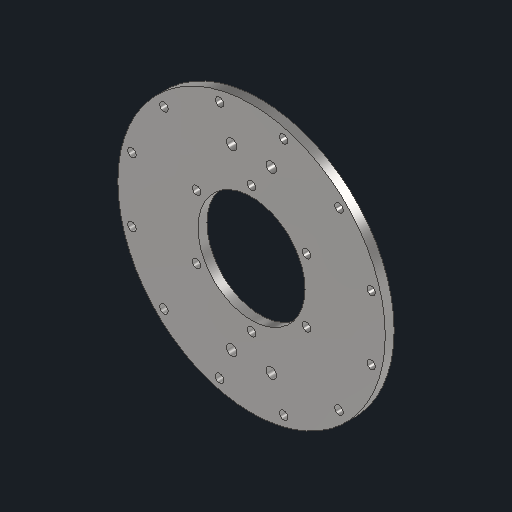
# Autodesk Inventor part: scara-plate1
Saved by Autodesk Inventor 2022 (Build 260153000, 153)
## iProperties
Created: 2021-10-10
Part Number: scara-plate1
Material: 鋼、炭素鋼
Document SubType Name: Sheet Metal
Designer: Yuta Kage
Density: 7.85 g/cm^3
Sheet Metal Rule: Default
Appearance: 半つや出し
Description: 在庫有
Author: Yuta Kage
Autodesk Inventor part; units mm, degrees
ref_plane "YZ Plane" through (0, 0, 0) normal (1, 0, 0) x (0, 1, 0)
ref_plane "XZ Plane" through (0, 0, 0) normal (0, 1, 0) x (-1, 0, 0)
ref_plane "XY Plane" through (0, 0, 0) normal (0, 0, 1) x (1, 0, 0)
sketch "スケッチ1" plane through (0, 0, 0) normal (0, 0, 1) x (1, 0, 0)
  line L0 (-20, -100) -> (20, -100)
  circle A0 centre (0, 0) radius 67.5
  dimension "d47" = 135
  constraints: 2 end point, 1 centre point, 1 coincident, 1 horizontal
  measures "d47" diameter of A0
extrude "プレート1" add sketch "スケッチ1" along normal blind 4.5
sketch "スケッチ2" plane through (0, 0, 4.5) normal (0, 0, 1) x (1, 0, 0)
  circle A0 centre (0, 0) radius 62.5
  point P0 (-44.1942, -44.1942)
  point P1 (-16.1762, -60.3704)
  point P2 (16.1762, -60.3704)
  point P3 (44.1942, -44.1942)
  point P4 (60.3704, -16.1762)
  point P5 (60.3704, 16.1762)
  point P6 (44.1942, 44.1942)
  point P7 (16.1762, 60.3704)
  point P8 (-16.1762, 60.3704)
  point P9 (-44.1942, 44.1942)
  point P10 (-60.3704, 16.1762)
  point P11 (-60.3704, -16.1762)
  dimension "d5" = 125
  dimension "d8" = 360
  dimension "d51" = 0
  constraints: 1 coincident, 16 other
  measures "d51" vertical distance of point (16.176, 60.37) point (-16.176, 60.37)
hole "穴1" at (-60.3704, -16.1762, 4.5) at (-60.3704, 16.1762, 4.5) at (-44.1942, 44.1942, 4.5) at (-16.1762, 60.3704, 4.5) at (16.1762, 60.3704, 4.5) at (44.1942, 44.1942, 4.5) at (60.3704, 16.1762, 4.5) at (60.3704, -16.1762, 4.5) at (44.1942, -44.1942, 4.5) at (16.1762, -60.3704, 4.5) at (-16.1762, -60.3704, 4.5) at (-44.1942, -44.1942, 4.5) direction (0, 0, -1) diameter 4.3 end through all clearance for "Socket Head Cap Screw" size "M4" standard "Ansi Metric M Profile"
sketch "スケッチ3" plane through (0, 0, 4.5) normal (0, 0, 1) x (1, 0, 0)
  circle A0 centre (0, 0) radius 27
  dimension "d18" = 54
  constraints: 1 centre point, 1 coincident
  measures "d18" diameter of A0
extrude "押し出し1" cut sketch "スケッチ3" against normal blind 10
sketch "スケッチ4" plane through (0, 0, 4.5) normal (0, 0, 1) x (1, 0, 0)
  line L0 (10, -45) -> (-10, -45)
  line L1 (-10, -45) -> (-10, 45)
  line L2 (-10, 45) -> (10, 45)
  line L3 (10, 45) -> (10, -45)
  line L4 (10, -45) -> (-10, 45) construction
  line L5 (-10, -45) -> (10, 45) construction
  circle A0 centre (0, 0) radius 45.5
  point P0 (0, 0)
  point P1 (0, 0)
  dimension "d21" = 20
  dimension "d46" = 91
  dimension "d48" = 90
  constraints: 12 end point, 4 midpoint, 3 coincident, 2 parallel, 1 centre point, 1 horizontal, 1 perpendicular
  measures "d21" distance of L1.end L2.end
  measures "d46" diameter of A0
  measures "d48" distance of L2.end L0.start
hole "穴2" at (-10, 45, 4.5) at (10, 45, 4.5) at (-10, -45, 4.5) at (10, -45, 4.5) direction (0, 0, -1) diameter 5.3 end through all clearance for "Socket Head Cap Screw" size "M5" standard "Ansi Metric M Profile"
sketch "スケッチ5" plane through (0, 0, 4.5) normal (0, 0, 1) x (1, 0, 0)
  circle A0 centre (0, 0) radius 32
  point P0 (0, 32)
  point P1 (-27.7128, 16)
  point P2 (-27.7128, -16)
  point P3 (0, -32)
  point P4 (27.7128, -16)
  point P5 (27.7128, 16)
  dimension "d33" = 64
  dimension "d36" = 360
  dimension "d49" = 0
  constraints: 1 coincident, 1 vertical alignment, 9 other
  measures "d49" horizontal distance of point (0, -32) point (0, 32)
hole "穴3" at (0, 32, 4.5) at (-27.7128, 16, 4.5) at (-27.7128, -16, 4.5) at (0, -32, 4.5) at (27.7128, -16, 4.5) at (27.7128, 16, 4.5) direction (0, 0, -1) diameter 4.3 end through all clearance for "Socket Head Cap Screw" size "M4" standard "Ansi Metric M Profile"
equation "\"d16\" = Thickness"
equation "\"d44\" = Thickness"
equation "\"d3\" = Thickness"
equation "\"BendRadius\" = Thickness"
equation "\"BendReliefWidth\" = Thickness"
equation "\"BendReliefDepth\" = 0.5 * Thickness"
equation "\"CornerReliefSize\" = 4 * Thickness"
equation "\"MinimumRemnant\" = 2 * Thickness"
equation "\"TransitionRadius\" = BendRadius"
equation "\"JacobiRadiusSize\" = BendRadius"
equation "\"GapSize\" = Thickness"
equation "\"Thickness\" = 4.5"
